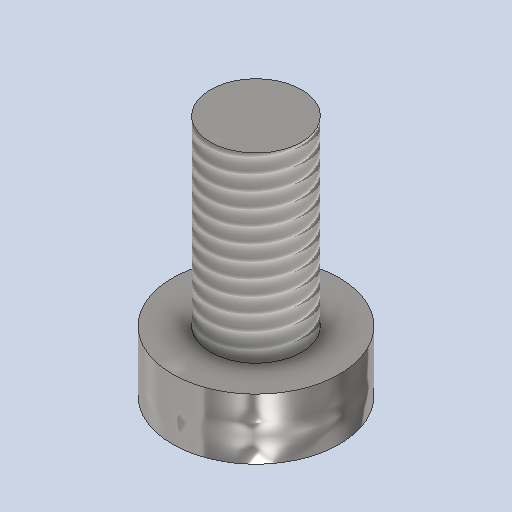
# Autodesk Inventor part: ULC-0306
Saved by Autodesk Inventor 2024.2 (Build 282272000, 272)
## iProperties
Created: 2024-01-03
Part Number: ULC-0306
Material: Stainless Steel AISI 304
Document SubType Name: Modeling
Designer: Masato Kubotera
Density: 8 g/cm^3
Appearance: Satin Hammered
Vendor: NISSAN SCREW
Mass: 0.677855 g
Surface Area: 1.49015 cm^2
Volume: 0.0847319 cm^3
Catalog Web Link: https://wilco.jp/products/U/ULC.html#page1
Author: Masato Kubotera
Autodesk Inventor part; units mm, degrees
ref_plane "YZ Plane" through (0, 0, 0) normal (1, 0, 0) x (0, 1, 0)
ref_plane "XZ Plane" through (0, 0, 0) normal (0, 1, 0) x (-1, 0, 0)
ref_plane "XY Plane" through (0, 0, 0) normal (0, 0, 1) x (1, 0, 0)
sketch "Sketch1" plane through (0, 0, 0) normal (0, 1, 0) x (-1, 0, 0)
  line L0 (0, 0) -> (-2.75, 0)
  line L1 (-2.75, 0) -> (-2.75, 2)
  line L2 (-2.75, 2) -> (-1.5, 2)
  line L3 (-1.5, 2) -> (-1.5, 8)
  line L4 (-1.5, 8) -> (0, 8)
  line L5 (0, 8) -> (0, 0)
  dimension "ScrewLength" = 6
  dimension "Diameter" = 5.5
  dimension "Metric" = 3
  dimension "HeadLength" = 2
  constraints: 12 end point, 3 horizontal, 3 vertical
  measures "ScrewLength" distance of L2.end L3.end
  measures "Diameter" diameter of L1 L5
  measures "Metric" diameter of L3 L5
  measures "HeadLength" distance of L0.end L1.end
revolve "Revolution1" add sketch "Sketch1" angle 360 about axis through (0, 0, 8) along (0, 0, -1)
thread "Thread1" size "M3x0.5" class "6g" standard "ANSI Metric M Profile" full length
sketch "Sketch2" plane through (0, 0, 0) normal (0, 0, -1) x (-1, 0, 0)
  line L0 (0.5774, 1) -> (1.1547, 0)
  line L1 (1.1547, 0) -> (0.5774, -1)
  line L2 (0.5774, -1) -> (-0.5774, -1)
  line L3 (-0.5774, -1) -> (-1.1547, 0)
  line L4 (-1.1547, 0) -> (-0.5774, 1)
  line L5 (-0.5774, 1) -> (0.5774, 1)
  point P0 (0, 0)
  point P1 (0, 0)
  dimension "WidthAcrossFlat" = 2
  constraints: 12 end point, 1 coincident, 1 horizontal, 13 other
  measures "WidthAcrossFlat" distance between parallel lines of L2 L5
extrude "Extrusion1" cut sketch "Sketch2" against normal blind 1.5
body "Solid1"
